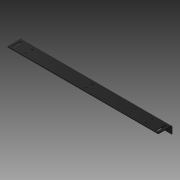
# Autodesk Inventor part: formed_right_left
Saved by Autodesk Inventor 2013 SP2 (Build 170200200, 200)
## iProperties
Created: 2013-05-31
Part Number: formed_right_left
Material: Steel, Mild
Document SubType Name: Sheet Metal
Designer: Edward
Density: 7.86 g/cm^3
Sheet Metal Rule: Default_mm
Flat Pattern Width: 6.57858 cm
Flat Pattern Length: 49 cm
Flat Pattern Area: 322.351 cm^2
Sheet Metal Width: 65.786 mm
Sheet Metal Length: 490.000 mm
Sheet Metal Area: 32235.062 mm^2
Vendor: custom
Description: formed side strap (16ga mild steel)
Mass: 753.394 g
Surface Area: 679.428 cm^2
Volume: 95.8517 cm^3
Stock Number: SM_LR
Author: Edward
Autodesk Inventor part; units mm, degrees
ref_plane "YZ Plane" through (0, 0, 0) normal (1, 0, 0) x (0, 1, 0)
ref_plane "XZ Plane" through (0, 0, 0) normal (0, 1, 0) x (-1, 0, 0)
ref_plane "XY Plane" through (0, 0, 0) normal (0, 0, 1) x (1, 0, 0)
sketch "Sketch1" plane through (0, 0, 0) normal (0, 0, 1) x (1, 0, 0)
  line L0 (-245, 20) -> (245, 20)
  line L1 (245, 20) -> (245, -20)
  line L2 (245, -20) -> (-245, -20)
  line L3 (-245, -20) -> (-245, 20)
  point P0 (0, 0)
  dimension "d0" = 490
  dimension "d1" = 40
  dimension "d2" = 20
  dimension "d3" = 245
  measures "d0" distance of L1.end L2.end
  measures "d1" distance of L0.end L1.end
  measures "d2" distance from line of L0 point (0, 0)
  measures "d3" distance from line of L3 point (0, 0)
extrude "Plate1" add sketch "Sketch1" along normal blind 3
sketch "Sketch2" plane through (0, 0, 3) normal (0, 0, 1) x (1, 0, 0)
  line L0 (-245, 20) -> (245, 20) projected
  line L1 (-245, -20) -> (-245, 20) projected
  arc A0 (-232.25, 12.5) -> (-237.75, 12.5) centre (-235, 12.5) ccw
  arc A1 (-237.75, -12.5) -> (-232.25, -12.5) centre (-235, -12.5) ccw
  line L2 (-237.75, 12.5) -> (-237.75, -12.5)
  line L3 (-232.25, -12.5) -> (-232.25, 12.5)
  point P0 (0, 0)
  dimension "d5" = 5.5
  dimension "d6" = 5.5
  dimension "d8" = 10
  dimension "d9" = 10
  dimension "d11" = 7.5
  dimension "d27" = 25
  dimension "d28" = 25
  constraints: 4 end point, 4 point on circle, 3 tangent, 2 centre point
  measures "d5" diameter of A0
  measures "d6" diameter of A1
  measures "d8" distance from line of L1 A0.centre
  measures "d9" distance from line of L1 A1.centre
  measures "d11" distance from line of L0 A0.centre
  measures "d27" distance of A0.centre A1.centre
  measures "d28" distance of L2.start L2.end
extrude "Extrusion1" cut sketch "Sketch2" against normal blind 10
pattern_linear "Rectangular Pattern1" count 2 spacing 470 along (1, 0, 0) of "Extrusion1"
sketch "Sketch3" plane through (245, 23, -3) normal (0, 1, 0) x (-1, 0, 0)
  line L0 (490, 0) -> (0, 0)
  line L1 (0, 0) -> (0, -19)
  line L2 (0, -19) -> (490, -19)
  line L3 (490, -19) -> (490, 0)
  constraints: 6 end point, 1 horizontal, 1 perpendicular, 1 vertical
edge flange "Flange1" height 25 angle 90 thickness 3 bend radius 3 thickness toward (0, 1, 0) relief tear relief width 3 relief depth 1.5 edges at (0, 20, 0) wall of the first edge with corners at (-245, 23, -3) (245, 23, -3) (245, 23, -22) (-245, 23, -22)
bend "Bend1"
corner "Corner1"
sketch "Sketch4" plane through (-245, 26, -22) normal (0, 1, 0) x (1, 0, 0)
  line L0 (0, 0) -> (490, 0) projected
  line L1 (0, -19) -> (0, 0) projected
  circle A0 centre (10, -9.5) radius 2
  circle A1 centre (110, -9.5) radius 2
  point P0 (245, -22)
  dimension "d29" = 4
  dimension "d30" = 9.5
  dimension "d31" = 10
  dimension "d32" = 4
  dimension "d33" = 110
  dimension "d34" = 9.5
  constraints: 2 centre point
  measures "d29" diameter of A0
  measures "d30" distance from line of L0 A0.centre
  measures "d31" distance from line of L1 A0.centre
  measures "d32" diameter of A1
  measures "d33" distance from line of L1 A1.centre
  measures "d34" distance from line of L0 A1.centre
extrude "Extrusion2" cut sketch "Sketch4" against normal through all
pattern_linear "Rectangular Pattern2" count 4 spacing 125 along (1, 0, 0) of "Extrusion2"
sketch "Sketch5" plane through (0, 0, 3) normal (0, 0, 1) x (1, 0, 0)
  line L0 (-245, 20) -> (245, 20) projected
  line L1 (-245, -20) -> (-245, 20) projected
  circle A0 centre (-195, 10) radius 2.75
  circle A1 centre (-195, -10) radius 2.75
  point P0 (0, 0)
  dimension "d40" = 5.5
  dimension "d41" = 5.5
  dimension "d42" = 20
  dimension "d43" = 10
  dimension "d44" = 50
  dimension "d45" = 50
  constraints: 2 centre point
  measures "d40" diameter of A0
  measures "d41" diameter of A1
  measures "d42" distance of A1.centre A0.centre
  measures "d43" distance from line of L0 A0.centre
  measures "d44" distance from line of L1 A0.centre
  measures "d45" distance from line of L1 A1.centre
extrude "Extrusion3" cut sketch "Sketch5" against normal through all
pattern_linear "Rectangular Pattern3" count 3 spacing 195 along (1, 0, 0) of "Extrusion3"
equation "\"d17\" = BendReliefWidth"
equation "\"d18\" = BendReliefDepth"
equation "\"d19\" = MinimumRemnant"
equation "\"d20\" = BendRadius"
equation "\"d23\" = BendRadius"
equation "\"d24\" = CornerReliefSize"
equation "\"d25\" = GapSize"
equation "\"d26\" = JacobiRadiusSize"
equation "\"d2\" = 0.5 * d1"
equation "\"d3\" = 0.5 * d0"
equation "\"BendRadius\" = Thickness"
equation "\"BendReliefWidth\" = Thickness"
equation "\"BendReliefDepth\" = 0.5 * Thickness"
equation "\"CornerReliefSize\" = 4 * Thickness"
equation "\"MinimumRemnant\" = 2 * Thickness"
equation "\"TransitionRadius\" = BendRadius"
equation "\"JacobiRadiusSize\" = BendRadius"
equation "\"GapSize\" = Thickness"
equation "\"d4\" = BendRadius"
equation "\"Thickness\" = 3"
body "Solid1"
